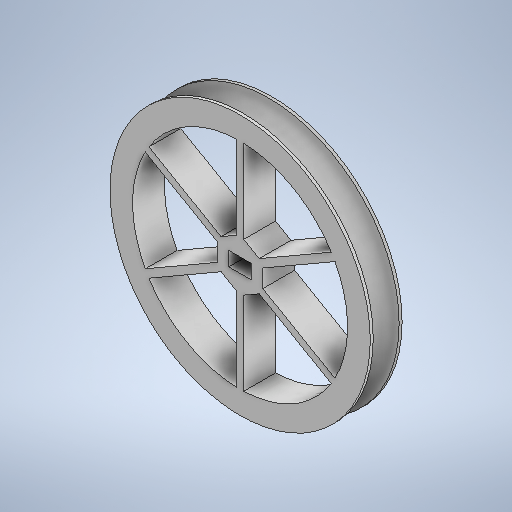
# Autodesk Inventor part: Wheel-D63C
Saved by Autodesk Inventor 2025.3 (Build 293356000, 356)
## iProperties
Created: 2025-09-04
Part Number: Wheel-D63C
Material: 一般
Document SubType Name: Modeling
Designer: daisuke
Density: 1 g/cm^3
Appearance: 既定
Author: daisuke
Autodesk Inventor part; units mm, degrees
ref_plane "YZ Plane" through (0, 0, 0) normal (1, 0, 0) x (0, 1, 0)
ref_plane "XZ Plane" through (0, 0, 0) normal (0, 1, 0) x (-1, 0, 0)
ref_plane "XY Plane" through (0, 0, 0) normal (0, 0, 1) x (1, 0, 0)
sketch "スケッチ1" plane through (0, 0, 0) normal (0, 1, 0) x (-1, 0, 0)
  line L0 (0, 0) -> (-64.0652, 0) construction
  circle A0 centre (-28.65, 0) radius 2.85
  line L1 (-23.65, -3.5) -> (-28.65, -3.5)
  line L2 (-28.65, -3.5) -> (-28.65, 3.5)
  line L3 (-28.65, 3.5) -> (-23.65, 3.5)
  line L4 (-23.65, 3.5) -> (-23.65, -3.5)
  line L5 (0, -4.9) -> (0, 4.9) projected
  point P0 (-28.65, 2.85)
  point P1 (-28.65, -2.85)
  dimension "P_DIA" = 5.7
  dimension "P_D1" = 28.65
  dimension "d2" = 7
  dimension "d3" = 5
  constraints: 10 end point, 2 horizontal, 2 parallel, 1 centre point, 1 midpoint, 1 perpendicular, 1 point on line
  measures "P_DIA" diameter of A0
  measures "P_D1" distance of A0.centre L0.start
  measures "d2" distance of L1.end L2.end
  measures "d3" distance of L1.start L1.end
revolve "リム" add sketch "スケッチ1" angle 360 about axis through (0, 0, -10) along (0, 0, 1) contours A0 L2 L3 L4 L1
sketch "スケッチ3" plane through (0, 0, 3.5) normal (0, 0, 1) x (1, 0, 0)
  line L0 (-5, 2.8868) -> (0, 5.7735)
  line L1 (0, 5.7735) -> (5, 2.8868)
  line L2 (5, 2.8868) -> (5, -2.8868)
  line L3 (5, -2.8868) -> (0, -5.7735)
  line L4 (0, -5.7735) -> (-5, -2.8868)
  line L5 (-5, -2.8868) -> (-5, 2.8868)
  point P0 (0, 0)
  point P1 (0, 0)
  dimension "HUB_DIA" = 10
  constraints: 12 end point, 1 coincident, 1 vertical alignment, 13 other
  measures "HUB_DIA" distance between parallel lines of L5 L2
extrude "ハブ" add sketch "スケッチ3" against normal up to surface (7 mm away)
sketch "スケッチ4" plane through (0, 0, 3.5) normal (0, 0, 1) x (1, 0, 0)
  line L0 (-0.8, 0) -> (0.8, 0)
  line L1 (0.8, 0) -> (0.8, 23.65)
  line L2 (0.8, 23.65) -> (-0.8, 23.65)
  line L3 (-0.8, 23.65) -> (-0.8, 0)
  circle A0 centre (0, 0) radius 23.65 projected
  point P0 (0, 23.65)
  dimension "SPOKE_THIN" = 1.6
  constraints: 8 end point, 2 midpoint, 2 parallel, 1 coincident, 1 horizontal, 1 perpendicular, 1 vertical alignment, 1 other
  measures "SPOKE_THIN" distance between parallel lines of L1 L3
extrude "スポーク" add sketch "スケッチ4" against normal up to surface (7 mm away) contours L3 A0 L1 L0 | L3 L2 A0 | A0 L2 L1 picked at (0, 7.8833)
pattern_circular "円形状パターン1" count 6 over 360 about axis through (0, 0, -10) along (0, 0, 1) of "スポーク"
sketch "スケッチ5" plane through (0, 0, 3.5) normal (0, 0, 1) x (1, 0, 0)
  line L0 (-2.5, 1.575) -> (2.5, 1.575)
  line L1 (2.5, 1.575) -> (2.5, -1.575)
  line L2 (2.5, -1.575) -> (-2.5, -1.575)
  line L3 (-2.5, -1.575) -> (-2.5, 1.575)
  point P0 (0, 0)
  point P1 (0, 1.575)
  point P2 (-2.5, 0)
  dimension "d15" = 5
  dimension "d16" = 3.15
  constraints: 8 end point, 2 midpoint, 2 parallel, 1 horizontal, 1 horizontal alignment, 1 perpendicular, 1 vertical alignment
  measures "d15" distance of L1.end L2.end
  measures "d16" distance of L0.end L1.end
extrude "軸穴" cut sketch "スケッチ5" against normal through all
